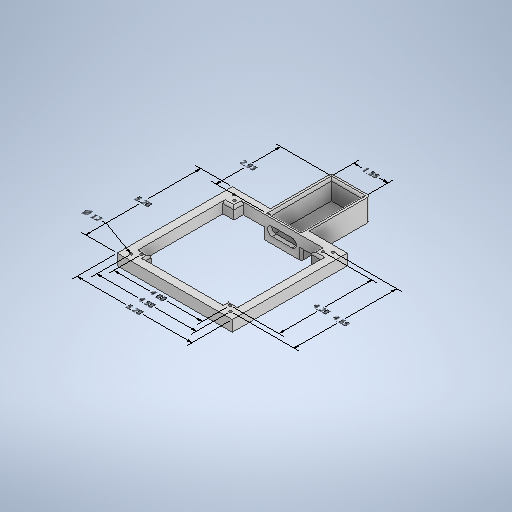
# Autodesk Inventor part: PCB_mount
Saved by Autodesk Inventor 2025.2 (Build 292293000, 293)
## iProperties
Created: 2025-04-17
Part Number: PCB_mount
Material: Generic
Document SubType Name: Modeling
Designer: 3lin2
Density: 1 g/cm^3
Appearance: Default
Author: 3lin2
Autodesk Inventor part; units mm, degrees
ref_plane "YZ Plane" through (0, 0, 0) normal (1, 0, 0) x (0, 1, 0)
ref_plane "XZ Plane" through (0, 0, 0) normal (0, 1, 0) x (-1, 0, 0)
ref_plane "XY Plane" through (0, 0, 0) normal (0, 0, 1) x (1, 0, 0)
sketch "Sketch1" plane through (0, 0, 0) normal (0, 1, 0) x (-1, 0, 0)
  line L0 (66.04, 66.04) -> (-66.04, 66.04)
  line L1 (-66.04, 66.04) -> (-66.04, -66.04)
  line L2 (-66.04, -66.04) -> (66.04, -66.04)
  line L3 (66.04, -66.04) -> (66.04, 66.04)
  point P0 (0, 0)
  dimension "d0" = 132.08
  dimension "d1" = 132.08
  dimension "d2" = 66.04
  dimension "d3" = 66.04
  constraints: 8 end point, 2 parallel, 1 horizontal, 1 perpendicular
  measures "d0" distance of L2.end L1.end
  measures "d1" distance of L1.end L0.end
  measures "d2" distance from line of L3 point (0, 0)
  measures "d3" distance from line of L2 point (0, 0)
extrude "Extrusion1" add sketch "Sketch1" along normal blind 12.7
sketch "Sketch2" plane through (0, 12.7, 0) normal (0, 1, 0) x (1, 0, 0)
  line L0 (-66.04, 66.04) -> (-66.04, -66.04) projected
  line L1 (66.04, -66.04) -> (66.04, 66.04) projected
  line L2 (66.04, 66.04) -> (-66.04, 66.04) projected
  circle A0 centre (-57.15, -59.055) radius 1.524
  circle A1 centre (-57.15, 59.055) radius 1.524
  circle A2 centre (57.15, 59.055) radius 1.524
  circle A3 centre (57.15, -59.055) radius 1.524
  point P0 (0, 0)
  dimension "d7" = 118.11
  dimension "d8" = 114.3
  dimension "d9" = 0
  dimension "d10" = 118.11
  dimension "d11" = 114.3
  dimension "d12" = 8.89
  dimension "d14" = 8.89
  dimension "d15" = 6.985
  dimension "d16" = 3.048
  dimension "d17" = 3.048
  dimension "d18" = 3.048
  dimension "d19" = 3.048
  constraints: 4 centre point, 4 coincident
  measures "d7" distance of point (-57.15, 59.055) point (-57.15, -59.055)
  measures "d8" distance of point (-57.15, -59.055) point (57.15, -59.055)
  measures "d9" horizontal distance of point (57.15, -59.055) point (57.15, 59.055)
  measures "d10" distance of point (57.15, -59.055) point (57.15, 59.055)
  measures "d11" distance of point (57.15, 59.055) point (-57.15, 59.055)
  measures "d12" distance from line of L0 point (-57.15, 59.055)
  measures "d14" distance from line of L1 point (57.15, 59.055)
  measures "d15" distance from line of L2 point (-57.15, 59.055)
  measures "d16" diameter of A0
  measures "d17" diameter of A1
  measures "d18" diameter of A2
  measures "d19" diameter of A3
extrude "Extrusion2" cut sketch "Sketch2" against normal blind 25.4
thread "Thread1" size "M3x0.5" class "6H" standard "ANSI Metric M Profile" full length
thread "Thread2" size "M3x0.5" class "6H" standard "ANSI Metric M Profile" full length
thread "Thread3" size "M3x0.5" class "6H" standard "ANSI Metric M Profile" full length
thread "Thread4" size "M3x0.5" class "6H" standard "ANSI Metric M Profile" full length
sketch "Sketch3" plane through (0, 12.7, 0) normal (0, 1, 0) x (1, 0, 0)
  circle A0 centre (-50.8, 53.34) radius 1.524
  circle A1 centre (50.8, 53.34) radius 1.524
  circle A2 centre (-50.8, -53.34) radius 1.524
  circle A3 centre (50.8, -53.34) radius 1.524
  line L0 (-66.04, 66.04) -> (-66.04, -66.04) projected
  line L1 (66.04, 66.04) -> (-66.04, 66.04) projected
  point P0 (0, 0)
  dimension "d30" = 3.048
  dimension "d31" = 3.048
  dimension "d32" = 3.048
  dimension "d33" = 3.048
  dimension "d34" = 101.6
  dimension "d35" = 101.6
  dimension "d36" = 106.68
  dimension "d37" = 106.68
  dimension "d38" = 0
  dimension "d39" = 0
  dimension "d40" = 15.24
  dimension "d41" = 12.7
  constraints: 4 centre point
  measures "d30" diameter of A0
  measures "d31" diameter of A1
  measures "d32" diameter of A2
  measures "d33" diameter of A3
  measures "d34" distance of A1.centre A0.centre
  measures "d35" distance of A3.centre A2.centre
  measures "d36" distance of A0.centre A2.centre
  measures "d37" distance of A3.centre A1.centre
  measures "d38" vertical distance of A1.centre A0.centre
  measures "d39" horizontal distance of A2.centre A0.centre
  measures "d40" distance from line of L0 A0.centre
  measures "d41" distance from line of A0.centre L1
extrude "Extrusion3" cut sketch "Sketch3" against normal blind 25.4
thread "Thread5" size "M3x0.5" class "6H" standard "ANSI Metric M Profile" full length
thread "Thread6" size "M3x0.5" class "6H" standard "ANSI Metric M Profile" full length
thread "Thread7" size "M3x0.5" class "6H" standard "ANSI Metric M Profile" full length
thread "Thread8" size "M3x0.5" class "6H" standard "ISO Metric profile" full length
sketch "Sketch4" plane through (0, 12.7, 0) normal (0, 1, 0) x (1, 0, 0)
  line L0 (-57.15, -48.7895) -> (57.15, -48.7895)
  line L1 (57.15, -48.7895) -> (57.15, 46.4605)
  line L2 (57.15, 46.4605) -> (-57.15, 46.4605)
  line L3 (-57.15, 46.4605) -> (-57.15, -48.7895)
  line L4 (-44.4732, -57.15) -> (44.4268, -57.15)
  line L5 (44.4268, -57.15) -> (44.4268, 57.15)
  line L6 (44.4268, 57.15) -> (-44.4732, 57.15)
  line L7 (-44.4732, 57.15) -> (-44.4732, -57.15)
  line L8 (66.04, 66.04) -> (-66.04, 66.04) projected
  point P0 (0, 0)
  point P1 (-44.4732, -48.7895)
  point P2 (44.4268, -48.7895)
  point P3 (44.4268, 46.4605)
  point P4 (-44.4732, 46.4605)
  dimension "d52" = 114.3
  dimension "d53" = 95.25
  dimension "d54" = 57.15
  dimension "d55" = 88.9
  dimension "d56" = 114.3
  dimension "d57" = 8.89
  constraints: 16 end point, 4 parallel, 2 horizontal, 2 perpendicular
  measures "d52" distance of L2.end L1.end
  measures "d53" distance of L1.end L0.end
  measures "d54" distance from line of L1 point (0, 0)
  measures "d55" distance of L6.end L5.end
  measures "d56" distance of L5.end L4.end
  measures "d57" distance between parallel lines of L8 L6
extrude "Extrusion4" cut sketch "Sketch4" against normal blind 25.4
sketch "Sketch5" plane through (66.04, 0, -66.04) normal (0, 0, -1) x (-1, 0, 0)
  line L0 (0, 0) -> (132.08, 0) projected
  line L1 (0, 12.7) -> (132.08, 12.7) projected
  line L2 (88.265, 0) -> (43.815, 0)
  line L3 (43.815, 0) -> (43.815, 12.7)
  line L4 (43.815, 12.7) -> (88.265, 12.7)
  line L5 (88.265, 12.7) -> (88.265, 0)
  line L6 (132.08, 0) -> (132.08, 12.7) projected
  point P0 (66.04, 0)
  point P1 (132.08, 6.35)
  point P2 (88.265, 12.7)
  point P3 (43.815, 0)
  dimension "d60" = 44.45
  dimension "d61" = 43.815
  constraints: 8 end point, 2 parallel, 2 point on line, 1 horizontal, 1 midpoint, 1 perpendicular
  measures "d60" distance of L3.end L4.end
  measures "d61" distance from line of point (132.08, 6.35) L5
extrude "Extrusion5" add sketch "Sketch5" along normal blind 69.85 contours L3 L1 L5 L0
sketch "Sketch6" plane through (0, 12.7, 0) normal (0, 1, 0) x (1, 0, 0)
  line L0 (22.225, 135.89) -> (-22.225, 135.89) projected
  line L1 (-44.4732, 57.15) -> (44.4268, 57.15) projected
  line L2 (22.225, 135.89) -> (-22.225, 135.89)
  line L3 (-22.225, 135.89) -> (-22.225, 57.15)
  line L4 (-22.225, 57.15) -> (22.225, 57.15)
  line L5 (22.225, 57.15) -> (22.225, 135.89)
  point P0 (0, 0)
  dimension "d64" = 44.45
  constraints: 8 end point, 2 parallel, 1 horizontal, 1 perpendicular, 1 point on line
  measures "d64" distance of L4.end L3.end
extrude "Extrusion6" add sketch "Sketch6" against normal blind 25.4
sketch "Sketch8" plane through (0, 12.7, 0) normal (0, 1, 0) x (1, 0, 0)
  line L0 (17.145, 131.1275) -> (-17.145, 131.1275)
  line L1 (-17.145, 131.1275) -> (-17.145, 61.9125)
  line L2 (-17.145, 61.9125) -> (17.145, 61.9125)
  line L3 (17.145, 61.9125) -> (17.145, 131.1275)
  line L4 (22.225, 66.04) -> (22.225, 135.89) projected
  line L5 (-22.225, 135.89) -> (22.225, 135.89) projected
  point P0 (0, 0)
  point P1 (22.225, 100.965)
  dimension "d74" = 34.29
  dimension "d75" = 69.215
  dimension "d76" = 5.08
  dimension "d77" = 4.7625
  constraints: 8 end point, 2 parallel, 1 horizontal, 1 midpoint, 1 perpendicular
  measures "d74" distance of L2.end L1.end
  measures "d75" distance of L2.end L0.start
  measures "d76" distance from line of point (22.225, 100.965) L3
  measures "d77" distance between parallel lines of L5 L0
extrude "Extrusion8" cut sketch "Sketch8" against normal blind 22.225
fillet "Fillet3" radius 2.54 16 edges at (22.225, 0, -135.89) (-22.225, 0, -135.89) (-22.225, -6.35, -57.15) (22.225, -6.35, -57.15) (0, 12.7, -131.1275) (-17.145, 12.7, -96.52) (17.145, 12.7, -96.52) (0, 12.7, -61.9125) (-50.8116, 12.7, -46.4605) (-44.4732, 12.7, -51.8052) (44.4268, 12.7, -51.8052) (50.7884, 12.7, -46.4605) (-50.8116, 12.7, 48.7895) (-44.4732, 12.7, 52.9698) (44.4268, 12.7, 52.9698) (50.7884, 12.7, 48.7895)
sketch "Sketch9" plane through (-47.0132, 12.7, -57.15) normal (0, 0, 1) x (1, 0, 0)
  line L0 (30.5032, -12.7) -> (63.5232, -12.7) construction
  line L1 (35.5832, -17.78) -> (58.4432, -17.78)
  line L2 (58.4432, -7.62) -> (35.5832, -7.62)
  arc A0 (35.5832, -7.62) -> (35.5832, -17.78) centre (35.5832, -12.7) ccw
  arc A1 (58.4432, -17.78) -> (58.4432, -7.62) centre (58.4432, -12.7) ccw
  point P0 (47.0132, -12.7)
  point P1 (47.0132, -12.7)
  dimension "d81" = 10.16
  dimension "d82" = 0
  dimension "d83" = 11.43
  constraints: 8 end point, 6 point on circle, 4 tangent, 2 centre point, 2 point on line, 1 horizontal, 1 midpoint, 1 parallel
  measures "d81" diameter of A1
  measures "d82" distance of point (47.013, -12.7) point (47.013, -12.7)
  measures "d83" distance of point (47.013, -12.7) A0.centre
extrude "Extrusion9" cut sketch "Sketch9" against normal blind 22.225
body "Solid1"
